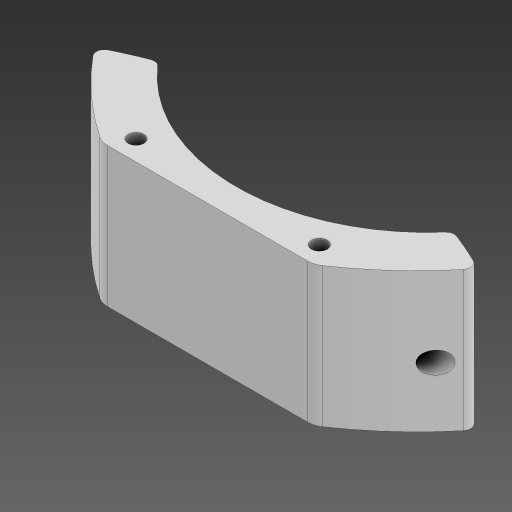
# Autodesk Inventor part: dribler_ball
Saved by Autodesk Inventor 2023 (Build 270158000, 158)
## iProperties
Created: 2025-06-23
Part Number: dribler_ball
Material: Типовые
Document SubType Name: Modeling
Designer: daa
Density: 1 g/cm^3
Appearance: По умолчанию
Author: daa
Autodesk Inventor part; units mm, degrees
ref_plane "YZ Plane" through (0, 0, 0) normal (1, 0, 0) x (0, 1, 0)
ref_plane "XZ Plane" through (0, 0, 0) normal (0, 1, 0) x (-1, 0, 0)
ref_plane "XY Plane" through (0, 0, 0) normal (0, 0, 1) x (1, 0, 0)
sketch "Эскиз1" plane through (0, 0, 0) normal (0, 1, 0) x (-1, 0, 0)
  line L0 (-25.0999, 67.4751) -> (25.1202, 67.4751)
  arc A0 (37.0101, 42.8778) -> (-36.9899, 42.8778) centre (0.0101, 12.3) ccw
  arc A1 (36.6633, -21.4663) -> (-36.0003, -21.4663) centre (0.3315, -28.4663) ccw
  line L1 (36.6633, -21.4663) -> (-36.0003, -21.4663)
  circle A2 centre (23.0101, 62.4751) radius 2
  arc A3 (37.0101, 42.8778) -> (48.0857, 47.7907) centre (0.4498, 140.2397) ccw
  circle A4 centre (-22.9899, 62.4751) radius 2
  arc A5 (-48.0655, 47.7901) -> (-36.9899, 42.8778) centre (-0.4338, 140.2412) ccw
  arc A6 (-27.9123, 66.6091) -> (-48.0655, 47.7901) centre (22.7111, -7.8037) ccw
  arc A7 (48.0857, 47.7907) -> (27.9326, 66.6092) centre (-22.6902, -7.8041) ccw
  arc A8 (27.9326, 66.6092) -> (25.1202, 67.4751) centre (25.1202, 62.4751) ccw
  arc A9 (-25.0999, 67.4751) -> (-27.9123, 66.6091) centre (-25.0999, 62.4751) ccw
  line L2 (37.0101, 42.8778) -> (-36.9899, 42.8778)
  point P0 (0, 0)
  point P1 (0, 0)
  point P2 (-26.6154, 67.4751)
  point P3 (0.0101, 60.3)
  point P4 (0.0102, 67.4751)
  point P5 (0, 0)
  point P6 (26.6357, 67.4751)
  point P7 (-26.5712, 67.2537)
  point P8 (26.5916, 67.2537)
  dimension "d0" = 72.6636
  dimension "d1" = 37
  dimension "d2" = 11.0756
  dimension "d3" = 7.1751
  dimension "d4" = 5
  dimension "d5" = 5
  dimension "d6" = 90
  dimension "d7" = 90
  dimension "d8" = 5
  dimension "d95" = 23
  dimension "d96" = 23
  dimension "d97" = 48
  dimension "d98" = 11.0756
  dimension "d105" = 74
  dimension "d107" = 4
  dimension "d108" = 4
  constraints: 21 point on circle, 10 centre point, 6 end point, 4 tangent, 3 horizontal, 2 point on line, 1 equal radius, 1 midpoint
  measures "d0" distance of L1.start L1.end
  measures "d1" radius of A1
  measures "d2" horizontal distance of A6.end L2.end
  measures "d3" distance of point (0.01, 67.475) point (0.01, 60.3)
  measures "d4" vertical distance of point (26.636, 67.475) A2.centre
  measures "d5" vertical distance of point (-26.615, 67.475) A4.centre
  measures "d6" radius of A6
  measures "d7" radius of A7
  measures "d8" radius of A8
  measures "d95" horizontal distance of point (0.01, 60.3) A2.centre
  measures "d96" horizontal distance of A4.centre point (0.01, 60.3)
  measures "d97" radius of A0
  measures "d98" horizontal distance of L2.start A7.start
  measures "d105" distance of L2.end L2.start
  measures "d107" diameter of A4
  measures "d108" diameter of A2
extrude "Выдавливание1" add sketch "Эскиз1" along normal blind 35 contours L0 A8 A7 A3 A0 A5 A6 A9
fillet "Сопряжение2" radius 2 4 edges at (48.0655, 17.5, 47.7901) (36.9899, 17.5, 42.8778) (-37.0101, 17.5, 42.8778) (-48.0857, 17.5, 47.7907)
ref_plane "РабПлоскость4" through (38.3242, 0, 43.3892) normal (0.3643311, 0, -0.9312695) x (0, 1, 0)
sketch "Эскиз9" plane through (38.3242, 0, 43.3892) normal (0.3643311, 0, -0.9312695) x (0, 1, 0)
  circle A0 centre (25, 3.3848) radius 2
  circle A1 centre (5, 3.3848) radius 2
  line L0 (35, 0) -> (35, 8.1748) projected
  line L1 (0, 8.1748) -> (35, 8.1748) projected
  point P0 (0, -51.4982)
  dimension "d49" = 4
  dimension "d50" = 4
  dimension "d51" = 20
  dimension "d52" = 10
  dimension "d53" = 4.79
  dimension "d54" = 4.79
  constraints: 2 centre point
  measures "d49" diameter of A0
  measures "d50" diameter of A1
  measures "d51" distance of A1.centre A0.centre
  measures "d52" distance from line of A0.centre L0
  measures "d53" distance from line of A0.centre L1
  measures "d54" distance from line of L1 A1.centre
extrude "Выдавливание6" cut sketch "Эскиз9" against normal blind 10
ref_plane "РабПлоскость9" through (-46.2409, 0, 45.7515) normal (0.4007186, 0, 0.9162012) x (0, -1, 0)
ref_plane "РабПлоскость8" through (-45.8402, 0, 46.6678) normal (0.4007186, 0, 0.9162012) x (0, -1, 0)
sketch "Эскиз12" plane through (-46.2409, 0, 45.7515) normal (0.4007186, 0, 0.9162012) x (0, -1, 0)
  circle A0 centre (-25, 3.3914) radius 2
  circle A1 centre (-5, 3.3914) radius 2
  line L0 (0, 8.1814) -> (-35, 8.1814) projected
  line L1 (-35, 8.1814) -> (-35, 0) projected
  point P0 (0, 60.6995)
  dimension "d66" = 4
  dimension "d67" = 4
  dimension "d68" = 20
  dimension "d69" = 4.79
  dimension "d70" = 4.79
  dimension "d71" = 10
  constraints: 2 centre point
  measures "d66" diameter of A0
  measures "d67" diameter of A1
  measures "d68" distance of A1.centre A0.centre
  measures "d69" distance from line of A0.centre L0
  measures "d70" distance from line of A1.centre L0
  measures "d71" distance from line of L1 A0.centre
extrude "Выдавливание8" cut sketch "Эскиз12" along normal blind 10
ref_plane "РабПлоскость12" through (46.4848, 0, 49.7456) normal (-0.9961947, 0, -0.0871557) x (0, -1, 0)
sketch "Эскиз14" plane through (46.4848, 0, 49.7456) normal (-0.9961947, 0, -0.0871557) x (0, -1, 0)
  circle A0 centre (-15, 4) radius 2.75
  line L0 (0, 18.418) -> (0, 0) projected
  line L1 (-35, 0) -> (0, 0) projected
  point P0 (0, -45.5049)
  dimension "d78" = 5.5
  dimension "d79" = 15
  dimension "d80" = 4
  constraints: 1 centre point
  measures "d78" diameter of A0
  measures "d79" distance from line of A0.centre L0
  measures "d80" distance from line of L1 A0.centre
extrude "Выдавливание9" cut sketch "Эскиз14" along normal blind 43.25
ref_plane "РабПлоскость13" through (-46.505, 0, 49.7461) normal (-0.9979898, 0, 0.0633754) x (0, 1, 0)
sketch "Эскиз16" plane through (-46.505, 0, 49.7461) normal (-0.9979898, 0, 0.0633754) x (0, 1, 0)
  circle A0 centre (15, -4) radius 2.25
  line L0 (0, -18.0062) -> (0, 0) projected
  line L1 (0, 0) -> (35, 0) projected
  point P0 (0, 46.6988)
  dimension "d85" = 4.5
  dimension "d86" = 15
  dimension "d87" = 4
  constraints: 1 centre point
  measures "d85" diameter of A0
  measures "d86" distance from line of L0 A0.centre
  measures "d87" distance from line of A0.centre L1
extrude "Выдавливание10" cut sketch "Эскиз16" against normal blind 15.5
sketch "Эскиз17" plane through (-46.505, 0, 49.7461) normal (-0.9979898, 0, 0.0633754) x (0, 1, 0)
  circle A0 centre (15, -4) radius 1.25
  line L0 (0, -18.0062) -> (0, 0) projected
  line L1 (0, 0) -> (35, 0) projected
  point P0 (0, 46.6988)
  dimension "d90" = 2.5
  dimension "d91" = 15
  dimension "d92" = 4
  constraints: 1 centre point
  measures "d90" diameter of A0
  measures "d91" distance from line of L0 A0.centre
  measures "d92" distance from line of A0.centre L1
extrude "Выдавливание11" cut sketch "Эскиз17" against normal blind 31.25
